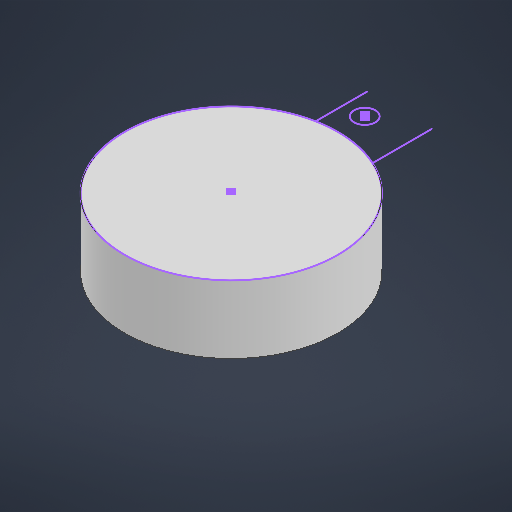
# Autodesk Inventor part: ball_caster
Saved by Autodesk Inventor 2026 (Build 300175050, 175E)
## iProperties
Created: 2025-06-14
Part Number: ball_caster
Material: Generic
Document SubType Name: Modeling
Designer: satom
Density: 1 g/cm^3
Appearance: Default
Author: satom
Autodesk Inventor part; units mm, degrees
ref_plane "YZ Plane" through (0, 0, 0) normal (1, 0, 0) x (0, 1, 0)
ref_plane "XZ Plane" through (0, 0, 0) normal (0, 1, 0) x (-1, 0, 0)
ref_plane "XY Plane" through (0, 0, 0) normal (0, 0, 1) x (1, 0, 0)
sketch "Sketch1" plane through (0, 0, 0) normal (0, 0, 1) x (1, 0, 0)
  line L0 (0, 0) -> (16, 0)
  line L1 (16, 0) -> (16, -10.16)
  line L2 (0, 0) -> (0, -20)
  arc A0 (0, -20) -> (5.3946, -14.6054) centre (0, -14.6054) ccw
  line L3 (0, -14.6054) -> (5.3946, -14.6054) construction
  line L4 (0, -14.6054) -> (0, -20) construction
  line L5 (5.3946, -14.6054) -> (16, -10.16)
  dimension "d0" = 16
  dimension "d1" = 20
  dimension "d2" = 10.16
  dimension "d3" = 90
  dimension "d4" = 5.3946
  constraints: 12 end point, 2 point on circle, 1 centre point, 1 horizontal, 1 perpendicular, 1 point on line, 1 vertical
  measures "d0" distance of L0.start L0.end
  measures "d1" distance of L0.start L2.end
  measures "d2" distance of L0.end L1.end
  measures "d3" angle of L4 L3
  measures "d4" radius of A0
revolve "Revolution1" add sketch "Sketch1" angle 360 about axis through (0, 0, 0) along (0, -1, 0)
sketch "Sketch2" plane through (0, 0, 0) normal (0, 1, 0) x (1, 0, 0)
  circle A0 centre (0, 0) radius 16
  line L0 (-3.0377, 23.4298) -> (-3.0377, 15.709)
  line L1 (6.6729, 14.5421) -> (6.6729, 23.4298)
  circle A1 centre (0, 20.0436) radius 1.5836
  constraints: 4 end point, 2 centre point, 2 point on circle, 2 vertical
body "Solid1"
